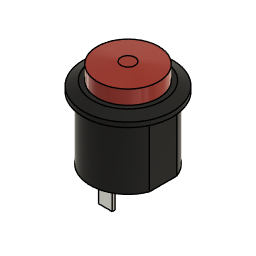
16mm button (Autodesk Fusion 360 design; units mm, degrees)
Autodesk Fusion 360 part; units mm, degrees
sketch "Sketch1" plane through (0, 0, 0) normal (0, 0, 1) x (1, 0, 0)
  circle A0 centre (0, 0) radius 8
  line L0 (7.45, -9) -> (-7.45, -9)
  line L1 (-7.45, -9) -> (-7.45, 9)
  line L2 (-7.45, 9) -> (7.45, 9)
  line L3 (7.45, 9) -> (7.45, -9)
  line L4 (7.45, -9) -> (-7.45, 9) construction
  line L5 (-7.45, -9) -> (7.45, 9) construction
  dimension "d1" = 16
  dimension "d2" = 14.9
  constraint coincident A0.centre origin
  constraint horizontal L0
  constraint perpendicular L0 L1
  constraint parallel L0 L2
  constraint parallel L1 L3
  constraint coincident L4 A0.centre
  constraint coincident L5 A0.centre
  measures "d1" diameter of A0
  measures "d2" distance of L1.end L2.end
extrude "Extrude1" add sketch "Sketch1" along normal blind 13.3 contours A0 L1 L3
sketch "Sketch2" plane through (0, 0, 13.3) normal (0, 0, 1) x (-1, 0, 0)
  arc A0 (7.45, 2.915) -> (-7.45, 2.915) centre (0, 0) ccw
  line L0 (-7.45, 2.915) -> (-7.45, -2.915)
  arc A1 (-7.45, -2.915) -> (7.45, -2.915) centre (0, 0) ccw
  line L1 (7.45, -2.915) -> (7.45, 2.915)
  circle A2 centre (0, 0) radius 9.45
  dimension "d5" = 18.9
  constraint concentric A0 A2
  measures "d5" diameter of A2
extrude "Extrude2" add sketch "Sketch2" along normal blind 2 contours A0 L0 A1 L1 | A2
chamfer "Chamfer1" distance 2 distance2 1 1 edges at (8.8105, 3.4173, 15.3) measured on face at (-3.5181, 1.5655, 15.3)
sketch "Sketch3" plane through (0, 0, 15.3) normal (0, 0, 1) x (-1, 0, 0)
  circle A0 centre (0, 0) radius 7.45
  circle A1 centre (0, 0) radius 6.5
  dimension "d10" = 13
  constraint coincident A0.centre A1.centre
  measures "d10" diameter of A1
extrude "Extrude3" add sketch "Sketch3" along normal blind 3.5 contours A1
chamfer "Chamfer2" distance 5 distance2 0.5 1 edges at (6.0601, 2.3505, 18.8) measured on face at (-1.9521, 0.9401, 18.8)
sketch "Sketch4" plane through (0, 0, 0) normal (0, 0, -1) x (1, 0, 0)
  arc A0 (7.45, 2.915) -> (-7.45, 2.915) centre (0, 0) ccw
  line L0 (-7.45, 2.915) -> (-7.45, -2.915)
  arc A1 (-7.45, -2.915) -> (7.45, -2.915) centre (0, 0) ccw
  line L1 (7.45, -2.915) -> (7.45, 2.915)
  line L2 (0, 8) -> (0, 4.8) construction
  line L3 (0, -8) -> (0, -4.8) construction
  line L4 (0, -4.8) -> (0, -4.2) construction
  line L5 (0, 4.8) -> (0, 4.2) construction
  line L6 (1.45, 4.2) -> (-1.45, 4.2)
  line L7 (-1.45, 4.2) -> (-1.45, 4.8)
  line L8 (-1.45, 4.8) -> (1.45, 4.8)
  line L9 (1.45, 4.8) -> (1.45, 4.2)
  line L10 (1.45, 4.2) -> (-1.45, 4.8) construction
  line L11 (-1.45, 4.2) -> (1.45, 4.8) construction
  line L12 (1.45, -4.8) -> (-1.45, -4.8)
  line L13 (-1.45, -4.8) -> (-1.45, -4.2)
  line L14 (-1.45, -4.2) -> (1.45, -4.2)
  line L15 (1.45, -4.2) -> (1.45, -4.8)
  line L16 (1.45, -4.8) -> (-1.45, -4.2) construction
  line L17 (-1.45, -4.8) -> (1.45, -4.2) construction
  point P0 (0, 4.5)
  point P1 (0, -4.5)
  dimension "d15" = 3.2
  dimension "d16" = 3.2
  dimension "d17" = 0.6
  dimension "d18" = 0.6
  dimension "d19" = 2.9
  dimension "d20" = 0.6
  dimension "d21" = 2.9
  dimension "d22" = 0.6
  constraint midpoint A0 L2.start
  constraint vertical L2
  constraint midpoint A1 L3.start
  constraint vertical L3
  constraint parallel L3 L4
  constraint parallel L2 L5
  constraint horizontal L6
  constraint perpendicular L6 L7
  constraint parallel L6 L8
  constraint parallel L7 L9
  constraint coincident L10 P0
  constraint coincident L11 P0
  constraint midpoint L5 P0
  constraint horizontal L12
  constraint perpendicular L12 L13
  constraint parallel L12 L14
  constraint parallel L13 L15
  constraint coincident L16 P1
  constraint coincident L17 P1
  constraint midpoint L4 P1
  measures "d15" distance of L2.start L2.end
  measures "d16" distance of L3.start L3.end
  measures "d17" distance of L3.end L4.end
  measures "d18" distance of L2.end L5.end
  measures "d19" distance of L7.end L8.end
  measures "d20" distance of L6.end L7.end
  measures "d21" distance of L13.end L14.end
  measures "d22" distance of L12.end L13.end
extrude "Extrude4" add sketch "Sketch4" along normal blind 5.7 contours L6 L7 L8 L9 | L12 L13 L14 L15
